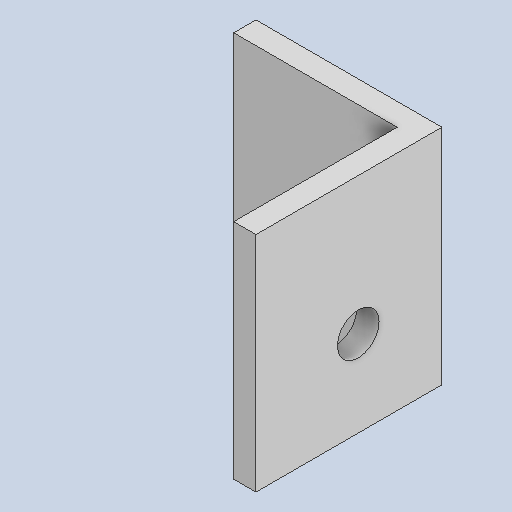
# Autodesk Inventor part: connector
Saved by Autodesk Inventor 2023.2 (Build 272271030, 271C)
## iProperties
Created: 2023-03-29
Part Number: connector
Material: Generic
Document SubType Name: Modeling
Designer: kao91
Density: 1 g/cm^3
Appearance: Default
Author: kao91
Autodesk Inventor part; units mm, degrees
ref_plane "YZ Plane" through (0, 0, 0) normal (1, 0, 0) x (0, 1, 0)
ref_plane "XZ Plane" through (0, 0, 0) normal (0, 1, 0) x (-1, 0, 0)
ref_plane "XY Plane" through (0, 0, 0) normal (0, 0, 1) x (1, 0, 0)
sketch "Sketch1" plane through (0, 0, 0) normal (0, 1, 0) x (-1, 0, 0)
  line L0 (0, 0) -> (-25, 0)
  line L1 (-25, 0) -> (-25, 3)
  line L2 (-25, 3) -> (0, 3)
  line L3 (0, 3) -> (0, 0)
  line L4 (-25, 0) -> (-22, 0)
  line L5 (-22, 0) -> (-22, 25)
  line L6 (-22, 25) -> (-25, 25)
  line L7 (-25, 25) -> (-25, 0)
  point P0 (0, 1.5)
  point P1 (-22, 3)
  dimension "d0" = 3
  dimension "d1" = 25
  dimension "d2" = 3
  dimension "d3" = 25
  constraints: 16 end point, 4 parallel, 2 horizontal, 2 perpendicular, 1 midpoint
  measures "d0" distance between parallel lines of L2 L0
  measures "d1" distance from line of point (0, 1.5) L1
  measures "d2" distance between parallel lines of L5 L1
  measures "d3" distance between parallel lines of L0 L6
extrude "Extrusion1" add sketch "Sketch1" along normal blind 30
sketch "Sketch2" plane through (22, 0, 3) normal (-1, 0, 0) x (0, 0, 1)
  circle A0 centre (8.25, 11.5611) radius 2.8 projected
  circle A1 centre (17, 32.0611) radius 1.5 projected
  circle A2 centre (-0.5, 32.0611) radius 1.5 projected
  point P0 (-3, 0)
extrude "Extrusion2" cut sketch "Sketch2" against normal blind 30
body "Solid1"
